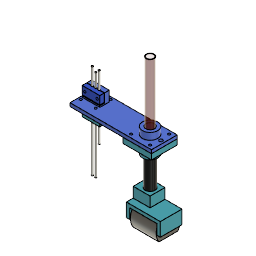
drain_box_parts (Autodesk Fusion 360 design; units mm, degrees)
Autodesk Fusion 360 part; units mm, degrees
sketch "top" plane through (0, 0, 0) normal (0, 0, 1) x (1, 0, 0) in component "pump_assy v1"
  line L0 (-19, 18) -> (19, 18) construction
  line L1 (19, 18) -> (19, -18) construction
  line L2 (19, -18) -> (-19, -18) construction
  line L3 (-19, -18) -> (-19, 18) construction
  circle A0 centre (-11, 2) radius 6
  line L4 (-19, -9) -> (-35, -9) construction
  line L5 (-35, -9) -> (-35, 1) construction
  line L6 (-35, 1) -> (-19, 1) construction
  line L7 (-19, 1) -> (-19, -9) construction
  circle A1 centre (-11, 2) radius 5
  dimension "d1" = 38
  dimension "d2" = 36
  dimension "d3" = 12
  dimension "d4" = 20
  dimension "d5" = 8
  dimension "d6" = 16
  dimension "d7" = 10
  dimension "d8" = 9
  dimension "d9" = 10
  constraint horizontal L0
  constraint vertical L1
  constraint horizontal L2
  constraint vertical L3
  constraint horizontal L4
  constraint vertical L5
  constraint horizontal L6
  constraint vertical L7
  constraint coincident L3 L4.start
  constraint concentric A0 A1
  measures "d1" distance of L0.start L0.end
  measures "d2" distance of L0.start L2.end
  measures "d3" diameter of A0
  measures "d4" distance of L2 A0.centre
  measures "d5" distance of L3 A0.centre
  measures "d6" distance of L4.start L4.end
  measures "d7" distance of L4.start L6.end
  measures "d8" distance of L2.end L4.start
  measures "d9" diameter of A1
sketch "center" plane through (0, 0, 0) normal (1, 0, 0) x (0, 1, 0) in component "pump_assy v1"
  line L0 (17, -13) -> (-19, -13)
  line L1 (-19, -13) -> (-19, 13) construction
  line L2 (-19, 13) -> (17, 13)
  line L3 (17, 13) -> (17, -13) construction
  line L4 (13, -13) -> (-15, -13) construction
  line L5 (-15, -13) -> (-15, 13) construction
  line L6 (-15, 13) -> (13, 13) construction
  line L7 (13, 13) -> (13, -13) construction
  arc A0 (13, -13) -> (13, 13) centre (-6.125, 0) ccw
  arc A1 (-15, 13) -> (-15, -13) centre (4.125, 0) ccw
  circle A2 centre (-4, 0) radius 5
  dimension "d10" = 36
  dimension "d11" = 26
  dimension "d12" = 10
  constraint horizontal L0
  constraint vertical L1
  constraint horizontal L2
  constraint vertical L3
  constraint horizontal L4
  constraint vertical L5
  constraint horizontal L6
  constraint vertical L7
  constraint coincident L2 L5.end
  constraint coincident L0 L4.start
  measures "d10" distance of L0.start L0.end
  measures "d11" distance of L0.start L2.end
  measures "d12" diameter of A2
extrude "Extrude1" add sketch "center" along normal blind -19 and the other way blind 35 contours A2 makes body 1 in component "pump_assy v1"
extrude "Extrude2" add sketch "top" along normal blind 33 and the other way blind -13 separate body contours A1 makes body 2 in component "pump_assy v1"
extrude "Extrude3" add sketch "top" along normal blind 18 and the other way blind -13 bodies 2 in component "pump_assy v1"
extrude "Extrude4" add sketch "center" along normal mid plane 38 contours L0 L2 A0 A1 | A2 bodies 1 2 in component "pump_assy v1"
extrude "Extrude5" add sketch "top" along normal blind 200 and the other way blind -18 separate body makes body 3 in component "pump_assy v1"
ref_plane "WorkPlane1" through (0, 0, 109) normal (0, 0, 1) x (1, 0, 0)
ref_plane "WorkPlane2" through (0, 0, 26) normal (0, 0, 1) x (1, 0, 0)
sketch "pump_top" plane through (0, 0, 26) normal (0, 0, 1) x (1, 0, 0)
  circle A0 centre (-11, 2) radius 5 construction
  circle A1 centre (-11, 2) radius 7.25
  line L0 (20, -19) -> (25, -19)
  line L1 (25, -19) -> (25, 13)
  line L2 (25, 13) -> (20, 13)
  line L3 (20, 13) -> (20, -19)
  line L4 (-25, -19) -> (-20, -19)
  line L5 (-20, -19) -> (-20, 13)
  line L6 (-20, 13) -> (-25, 13)
  line L7 (-25, 13) -> (-25, -19)
  line L8 (-20, -19) -> (20, -19)
  line L9 (-20, 13) -> (20, 13)
  circle A2 centre (-11, 2) radius 6.75
  line L10 (-25, -12) -> (-20, -12)
  line L11 (-25, 4) -> (-20, 4)
  line L12 (0, 13) -> (0, -9)
  line L13 (0, -9) -> (-25, -9)
  circle A3 centre (-11, 2) radius 6.5
  dimension "d34" = 14.5
  dimension "d35" = -0.5
  dimension "d67" = -0.75
  constraint concentric A0 A1
  constraint horizontal L0
  constraint vertical L1
  constraint horizontal L2
  constraint vertical L3
  constraint horizontal L4
  constraint vertical L5
  constraint horizontal L6
  constraint vertical L7
  constraint perpendicular L3 L8
  constraint perpendicular L3 L9
  constraint coincident L7 L10.start
  constraint coincident L5 L10.end
  constraint perpendicular L5 L10
  constraint coincident L7 L11.start
  constraint coincident L5 L11.end
  constraint perpendicular L5 L11
  constraint midpoint L9 L12.start
  constraint perpendicular L9 L12
  constraint coincident L7 L13.end
  constraint perpendicular L7 L13
  measures "d34" diameter of A1
sketch "inside_top" plane through (0, 0, 109) normal (0, 0, 1) x (1, 0, 0)
  circle A0 centre (-11, 2) radius 7.25
  circle A1 centre (-100, 6) radius 1.4
  circle A2 centre (-95, 6) radius 1.4
  circle A3 centre (-90, 6) radius 1.4
  line L0 (10, 21) -> (-32, 21)
  line L1 (-32, 21) -> (-32, -17)
  line L2 (-32, -17) -> (10, -17)
  line L3 (10, -17) -> (10, 21)
  line L4 (10, 21) -> (-32, -17) construction
  line L5 (-32, 21) -> (10, -17) construction
  line L6 (3, -12) -> (-25, -12) construction
  line L7 (-25, -12) -> (-25, 16) construction
  line L8 (-25, 16) -> (3, 16) construction
  line L9 (3, 16) -> (3, -12) construction
  line L10 (3, -12) -> (-25, 16) construction
  line L11 (-25, -12) -> (3, 16) construction
  circle A4 centre (-25, 16) radius 1.4
  circle A5 centre (-25, -12) radius 1.4
  circle A6 centre (3, -12) radius 1.4
  circle A7 centre (3, 16) radius 1.4
  circle A8 centre (-11, 2) radius 11.25
  line L12 (10, -17) -> (-110, -17) construction
  circle A9 centre (5, 2) radius 2.5
  line L13 (-32, 21) -> (-110, 21) construction
  line L14 (-110, 21) -> (-110, -17) construction
  line L15 (-110, 21) -> (-80, 21)
  line L16 (-80, 21) -> (-80, -9)
  line L17 (-80, -9) -> (-110, -9)
  line L18 (-110, -9) -> (-110, 21)
  circle A10 centre (-106, 17) radius 1.4
  circle A11 centre (-106, -5) radius 1.4
  circle A12 centre (-84, 17) radius 1.4
  circle A13 centre (-84, -5) radius 1.4
  line L19 (-108, 13) -> (-82, 13)
  line L20 (-82, 13) -> (-82, -1)
  line L21 (-82, -1) -> (-108, -1)
  line L22 (-108, -1) -> (-108, 13)
  circle A14 centre (-11, 2) radius 6.5
  circle A15 centre (-106, 17) radius 3 construction
  point P0 (-11, 2)
  point P1 (-11, 2)
  dimension "d37" = 2.8
  dimension "d38" = 2.8
  dimension "d39" = 2.8
  dimension "d40" = 42
  dimension "d41" = 38
  dimension "d42" = 28
  dimension "d43" = 28
  dimension "d44" = 2.8
  dimension "d45" = 2.8
  dimension "d46" = 2.8
  dimension "d47" = 2.8
  dimension "d48" = 4
  dimension "d49" = 120
  dimension "d51" = 5
  dimension "d52" = 2.8
  dimension "d53" = 2.8
  dimension "d54" = 2.8
  dimension "d55" = 2.8
  dimension "d56" = -0.75
  dimension "d86" = 6
  constraint horizontal L0
  constraint perpendicular L0 L1
  constraint parallel L0 L2
  constraint parallel L1 L3
  constraint coincident L4 P1
  constraint coincident L5 P1
  constraint coincident P0 A0.centre
  constraint horizontal L6
  constraint perpendicular L6 L7
  constraint parallel L6 L8
  constraint parallel L7 L9
  constraint coincident L10 P1
  constraint coincident L11 P1
  constraint coincident P1 P0
  constraint coincident L7.end L8.start
  constraint coincident L6.end L7.start
  constraint coincident L6.start L9.end
  constraint coincident L8.end L9.start
  constraint perpendicular L3 L12
  constraint perpendicular L1 L13
  constraint perpendicular L13 L14
  constraint horizontal L15
  constraint vertical L16
  constraint horizontal L17
  constraint vertical L18
  constraint horizontal L19
  constraint vertical L20
  constraint horizontal L21
  constraint vertical L22
  constraint concentric A10 A15
  measures "d37" diameter of A1
  measures "d38" diameter of A2
  measures "d39" diameter of A3
  measures "d40" distance of L1.end L2.end
  measures "d41" distance of L0.end L1.end
  measures "d42" distance of L7.end L8.end
  measures "d43" distance of L6.end L7.end
  measures "d44" diameter of A4
  measures "d45" diameter of A5
  measures "d46" diameter of A6
  measures "d47" diameter of A7
  measures "d49" distance of L2.end L12.end
  measures "d51" diameter of A9
  measures "d52" diameter of A10
  measures "d53" diameter of A11
  measures "d54" diameter of A12
  measures "d55" diameter of A13
  measures "d86" diameter of A15
sketch "outside_top" plane through (0, 0, 109) normal (0, 0, 1) x (1, 0, 0)
  circle A0 centre (-90, 6) radius 1.4
  circle A1 centre (-95, 6) radius 1.4
  circle A2 centre (-100, 6) radius 1.4
  circle A3 centre (-11, 2) radius 6.5
  circle A4 centre (5, 2) radius 2.5
  line L0 (-108, -1) -> (-108, 13)
  line L1 (-108, 13) -> (-82, 13)
  line L2 (-82, -1) -> (-108, -1)
  line L3 (-82, 13) -> (-82, -1)
  line L4 (-82, 6) -> (-108, 6)
  line L5 (-110, 21) -> (10, 21)
  line L6 (10, 21) -> (10, -17)
  line L7 (10, -17) -> (-110, -17)
  line L8 (-110, -17) -> (-110, 21)
  circle A5 centre (-11, 2) radius 11.25
  circle A6 centre (-106, 17) radius 1.7
  circle A7 centre (-84, 17) radius 1.7
  circle A8 centre (-106, -5) radius 1.7
  circle A9 centre (-84, -5) radius 1.7
  circle A10 centre (-25, 16) radius 1.7
  circle A11 centre (3, 16) radius 1.7
  circle A12 centre (-25, -12) radius 1.7
  circle A13 centre (3, -12) radius 1.7
  circle A14 centre (-11, 2) radius 7.25
  point P0 (-106, 17)
  point P1 (-84, 17)
  point P2 (-84, -5)
  point P3 (-106, -5)
  point P4 (-25, 16)
  point P5 (3, 16)
  point P6 (3, -12)
  point P7 (-25, -12)
  dimension "d87" = 3.4
  dimension "d88" = 3.4
  dimension "d89" = 3.4
  dimension "d90" = 3.4
  dimension "d93" = 3.4
  dimension "d94" = 3.4
  dimension "d95" = 3.4
  dimension "d96" = 3.4
  constraint midpoint L3 L4.start
  constraint midpoint L0 L4.end
  constraint horizontal L5
  constraint vertical L6
  constraint horizontal L7
  constraint vertical L8
  constraint coincident P0 A6.centre
  constraint coincident P1 A7.centre
  constraint coincident P3 A8.centre
  constraint coincident P2 A9.centre
  constraint coincident P4 A10.centre
  constraint coincident P5 A11.centre
  constraint coincident P7 A12.centre
  constraint coincident P6 A13.centre
  measures "d87" diameter of A6
  measures "d88" diameter of A7
  measures "d89" diameter of A8
  measures "d90" diameter of A9
  measures "d93" diameter of A10
  measures "d94" diameter of A11
  measures "d95" diameter of A12
  measures "d96" diameter of A13
extrude "Extrude2'" add sketch "pump_top" against normal blind 15 separate body contours L0 L1 L2 L3 | L4 L5 L7 L10 | L5 L6 L7 L11 makes body 4 at (-25, -14.3333, 21) makes body 5 at (-25, 7, 16) makes body 6 at (20, 2.3333, 21)
extrude "Extrude3'" add sketch "pump_top" against normal blind 4 contours L5 L7 L10 L13 | L5 L7 L11 L13 bodies 4 5
extrude "Extrude4'" add sketch "pump_top" along normal blind 20 contours L5 L9 L12 L13 | L5 L6 L7 L11 | L5 L7 L11 L13 bodies 4
extrude "Extrude5'" add sketch "pump_top" along normal blind 5 contours L0 L1 L2 L3 | L3 L5 L8 L9 L12 L13 | L4 L5 L7 L10 | L5 L7 L10 L13 bodies 4 6
extrude "Extrude6" add sketch "pump_top" along normal blind 2 contours A1 | A2 bodies 4
extrude "Extrude7" add sketch "inside_top" against normal blind 20 separate body contours A8 makes body 7
extrude "Extrude9" add sketch "inside_top" against normal blind 8 contours L0 L1 L2 L3 bodies 7
extrude "Extrude21" add sketch "inside_top" against normal blind 2 contours A0 bodies 7
extrude "Extrude10" add sketch "inside_top" against normal blind 8 separate body contours L15 L16 L17 L18 makes body 8
extrude "Extrude11" add sketch "inside_top" against normal blind 20 contours L19 L20 L21 L22 bodies 8
extrude "Extrude12" add sketch "outside_top" along normal blind 15 separate body contours A5 | A14 makes body 9
extrude "Extrude13" add sketch "outside_top" along normal blind 20 separate body contours A0 A1 A2 L0 L1 L3 L4 makes body 10
extrude "Extrude16" add sketch "outside_top" along normal blind 7 contours A0 A1 A2 L0 L2 L3 L4 bodies 10
extrude "Extrude17" add sketch "outside_top" along normal blind 5 contours L5 L6 L7 L8 bodies 9 10
extrude "Extrude15" add sketch "outside_top" along normal blind 5 contours A0 A1 A2 L0 L2 L3 L4 | L5 L6 L7 L8 bodies 9
extrude "Extrude18" add sketch "outside_top" along normal blind 20 and the other way blind -8 separate body contours A0 A1 A2 L0 L2 L3 L4 makes body 11
move_face "OffsetFaces1" offset -0.5 4 faces at (-84.2, 6, 121) (-92.1333, 6, 121) (-97.1333, 6, 121) (-103.6, 6, 121) on bodies 11
sketch "clamp_holes" plane through (0, -1, 0) normal (0, -1, 0) x (1, 0, 0)
  line L0 (-108, 129) -> (-82, 129) construction
  line L1 (-108, 117) -> (-108, 129) construction
  line L2 (-108, 117) -> (-82, 117) construction
  line L3 (-82, 117) -> (-82, 129) construction
  circle A0 centre (-104, 123) radius 1.7
  circle A1 centre (-104, 123) radius 1.4
  circle A2 centre (-86, 123) radius 1.7
  circle A3 centre (-86, 123) radius 1.4
  dimension "d108" = 3.4
  dimension "d109" = 2.8
  dimension "d110" = 3.4
  dimension "d111" = 2.8
  constraint concentric A0 A1
  constraint concentric A2 A3
  measures "d108" diameter of A0
  measures "d109" diameter of A1
  measures "d110" diameter of A2
  measures "d111" diameter of A3
extrude "Extrude19" cut sketch "clamp_holes" against normal blind 14 contours A1 | A3 bodies 9
extrude "Extrude20" cut sketch "clamp_holes" against normal blind 6.5 contours A0 | A1 | A2 | A3 bodies 11
extrude "Extrude22" add sketch "pump_top" along normal blind 80.5 and the other way blind -2.5 separate body contours A1 makes body 12
extrude "Extrude23" add sketch "inside_top" along normal blind -94 and the other way blind -45 separate body contours A1 makes body 13
extrude "Extrude24" add sketch "inside_top" along normal blind -94 and the other way blind -40 separate body contours A2 makes body 14
extrude "Extrude25" add sketch "inside_top" along normal blind -49 and the other way blind -45 separate body contours A3 makes body 15
extrude "Extrude26" add sketch "outside_top" along normal blind 1 separate body contours A0 A1 A2 L0 L2 L3 L4 | A0 A1 A2 L0 L1 L3 L4 | L5 L6 L7 L8 | A5 makes body 16
component "pump_assy v1" placed x (1, 0, 0) y (0, 1, 0) z (0, 0, 1) at (0, 0, 13)
hidden bodies 16
equation "depth = 109 mm"
equation "high = 60 mm"
equation "low = 15 mm"
equation "d8 = 15 mm - 6 mm"
equation "d13 = depth"
equation "cf_od = 14.5 mm"
equation "d34 = cf_od"
equation "rod_diam = 2.8 mm"
equation "d37 = rod_diam"
equation "d38 = rod_diam"
equation "d39 = rod_diam"
equation "d44 = screw_tight"
equation "d45 = screw_tight"
equation "d46 = screw_tight"
equation "d47 = screw_tight"
equation "d52 = screw_tight"
equation "d53 = screw_tight"
equation "d54 = screw_tight"
equation "d55 = screw_tight"
equation "d87 = screw_loose"
equation "d88 = screw_loose"
equation "d89 = screw_loose"
equation "d90 = screw_loose"
equation "screw_loose = 3.4 mm"
equation "screw_tight = 2.8 mm"
equation "d93 = screw_loose"
equation "d94 = screw_loose"
equation "d95 = screw_loose"
equation "d96 = screw_loose"
equation "d108 = screw_loose"
equation "d109 = screw_tight"
equation "d110 = screw_loose"
equation "d111 = screw_tight"
equation "d122 = -( depth - low )"
equation "d126 = -( depth - low )"
equation "d130 = -( depth - high )"
equation "cf_tube_length = 78 mm"
equation "low_rod = 140 mm"
equation "drive_rod = 135 mm"
equation "high_rod = 95 mm"
named bodies: "pump", "tube", "carbon_fiber_tube", "low_rod", "drive_rod", "high_rod", "hole_template"
